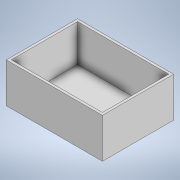
# Autodesk Inventor part: Case
Saved by Autodesk Inventor 2020 (Build 240168000, 168)
## iProperties
Created: 2019-09-29
Part Number: Case
Material: Generic
Document SubType Name: Modeling
Designer: bzs3334
Density: 1 g/cm^3
Appearance: Default
Author: bzs3334
Autodesk Inventor part; units mm, degrees
ref_plane "YZ Plane" through (0, 0, 0) normal (1, 0, 0) x (0, 1, 0)
ref_plane "XZ Plane" through (0, 0, 0) normal (0, 1, 0) x (-1, 0, 0)
ref_plane "XY Plane" through (0, 0, 0) normal (0, 0, 1) x (1, 0, 0)
sketch "Sketch1" plane through (0, 0, 0) normal (0, 1, 0) x (-1, 0, 0)
  line L0 (55, -40) -> (-55, -40)
  line L1 (-55, -40) -> (-55, 40)
  line L2 (-55, 40) -> (55, 40)
  line L3 (55, 40) -> (55, -40)
  line L4 (-58, -43) -> (58, -43)
  line L5 (58, -43) -> (58, 43)
  line L6 (58, 43) -> (-58, 43)
  line L7 (-58, 43) -> (-58, -43)
  point P0 (0, 0)
  dimension "d0" = 110
  dimension "d1" = 55
  dimension "d2" = 80
  dimension "d3" = 40
  dimension "d4" = 3
  constraints: 16 end point, 4 parallel, 2 perpendicular, 1 horizontal, 3 other
  measures "d0" distance of L0.start L0.end
  measures "d1" horizontal distance of L0.start point (0, 0)
  measures "d2" distance of L2.end L0.start
  measures "d3" vertical distance of L0.start point (0, 0)
  measures "d4" distance between parallel lines of L4 L0
extrude "Extrusion1" add sketch "Sketch1" against normal blind 3 contours L0 L1 L2 L3 | L7 L6 L5 L4
extrude "Extrusion2" add sketch "Sketch1" along normal blind 45
equation "\"d1\" = 0.5 * d0"
equation "\"d3\" = 0.5 * d2"
body "Solid1"
